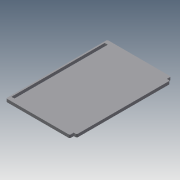
# Autodesk Inventor part: NewControlPanel
Saved by Autodesk Inventor 2014 (Build 180170000, 170)
## iProperties
Created: 2015-02-17
Part Number: NewControlPanel
Material: Generic
Document SubType Name: Modeling
Designer: Peele
Density: 1 g/cm^3
Appearance: Default
Author: Peele
Autodesk Inventor part; units mm, degrees
ref_plane "YZ Plane" through (0, 0, 0) normal (1, 0, 0) x (0, 1, 0)
ref_plane "XZ Plane" through (0, 0, 0) normal (0, 1, 0) x (-1, 0, 0)
ref_plane "XY Plane" through (0, 0, 0) normal (0, 0, 1) x (1, 0, 0)
sketch "Sketch1" plane through (0, 0, 0) normal (0, 0, 1) x (1, 0, 0)
  line L0 (0, 0) -> (128, 0)
  line L1 (128, 0) -> (128, 203.5927)
  line L2 (128, 203.5927) -> (0, 203.5927)
  line L3 (0, 203.5927) -> (0, 0)
  line L4 (0, 0) -> (-77.2375, 168.1052) construction
  line L5 (-77.2375, 168.1052) -> (0, 203.5927) construction
  line L6 (2.875, 195.5927) -> (9.125, 195.5927)
  line L7 (9.125, 195.5927) -> (9.125, 8)
  line L8 (9.125, 8) -> (2.875, 8)
  line L9 (2.875, 8) -> (2.875, 195.5927)
  dimension "d0" = 128
  dimension "d1" = 85
  dimension "d2" = 185
  dimension "d3" = 6.25
  dimension "d4" = 2.875
  dimension "d5" = 8
  dimension "d6" = 8
  constraints: 20 end point, 4 parallel, 3 perpendicular, 2 horizontal
  measures "d0" distance of L0.start L0.end
  measures "d1" distance from line of L2.end L4
  measures "d2" distance from line of L0.start L5
  measures "d3" distance of L6.start L6.end
  measures "d4" distance between parallel lines of L3 L9
  measures "d5" distance between parallel lines of L6 L2
  measures "d6" distance from line of L8.end L0
extrude "Extrusion1" add sketch "Sketch1" along normal blind 6
sketch "Sketch2" plane through (0, 0, 6) normal (0, 0, 1) x (1, 0, 0)
  line L0 (0, 0) -> (128, 0) projected
  line L1 (128, 0) -> (128, 203.5927) projected
  line L2 (128, 203.5927) -> (0, 203.5927) projected
  line L3 (128, 195.4927) -> (134, 195.4927)
  line L4 (134, 195.4927) -> (134, 8.1)
  line L5 (134, 8.1) -> (128, 8.1)
  line L6 (128, 8.1) -> (128, 195.4927)
  dimension "d9" = 8.1
  dimension "d10" = 8.1
  dimension "d11" = 6
  constraints: 8 end point, 2 parallel, 1 horizontal, 1 perpendicular, 1 point on line
  measures "d9" distance between parallel lines of L3 L2
  measures "d10" distance between parallel lines of L5 L0
  measures "d11" distance of L4.end L5.end
extrude "Extrusion2" add sketch "Sketch2" against normal blind 6
fillet "Fillet1" radius 2 6 edges at (134, 195.4927, 3) (128, 203.5927, 3) (0, 203.5927, 3) (128, 0, 3) (134, 8.1, 3) (0, 0, 3)
body "Solid1"
